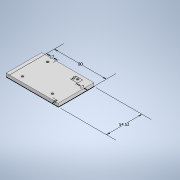
# Autodesk Inventor part: practica 13.2
Saved by Autodesk Inventor 2020.2 (Build 242310000, 310)
## iProperties
Created: 2020-02-28
Part Number: practica 13.2
Material: Genérico
Document SubType Name: Chapa
Designer: Luis Gallardo
Density: 1 g/cm^3
Sheet Metal Rule: Por defecto_mm
Appearance: Valor por defecto
Author: Luis Gallardo
Autodesk Inventor part; units mm, degrees
ref_plane "YZ Plane" through (0, 0, 0) normal (1, 0, 0) x (0, 1, 0)
ref_plane "XZ Plane" through (0, 0, 0) normal (0, 1, 0) x (-1, 0, 0)
ref_plane "XY Plane" through (0, 0, 0) normal (0, 0, 1) x (1, 0, 0)
sketch "Boceto1" plane through (0, 0, 0) normal (0, 1, 0) x (-1, 0, 0)
  line L0 (0, 0) -> (-80, 0)
  line L1 (-80, 0) -> (-80, -54.52)
  line L2 (-80, -54.52) -> (0, -54.52)
  line L3 (0, -54.52) -> (0, 0)
  line L4 (-80, -54.52) -> (-63, -54.52) construction
  line L5 (-63, -54.52) -> (-63, -46.52) construction
  line L6 (-63, 0) -> (-63, -8) construction
  line L7 (0, -54.52) -> (-17, -54.52) construction
  line L8 (-17, -54.52) -> (-17, -46.52) construction
  line L9 (-17, 0) -> (-17, -8) construction
  dimension "d0" = 80
  dimension "d1" = 54.52
  dimension "d2" = 17
  dimension "d3" = 8
  dimension "d6" = 8
  dimension "d7" = 17
  constraints: 20 end point, 6 perpendicular, 4 point on line, 1 horizontal, 1 parallel
  measures "d0" distance of L0.start L0.end
  measures "d1" distance of L0.end L1.end
  measures "d2" distance of L1.end L4.end
  measures "d3" distance of L4.end L5.end
  measures "d6" distance of L6.start L6.end
  measures "d7" distance of L2.end L7.end
extrude "Extrusión1" add sketch "Boceto1" along normal blind 5
hole "Agujero2" at (63, 0, -46.52) direction (0, 1, 0) diameter 3.242 end through all thread size "M4x0.7" class "6H" standard "ANSI Metric M Profile"
hole "Agujero3" at (17, 0, -46.52) at (63, 0, -8) at (17, 0, -8) direction (0, 1, 0) diameter 3.242 end through all thread size "M4x0.7" class "6H" standard "ANSI Metric M Profile"
equation "\"Radio_pliegue\" = Grosor"
equation "\"Anchura_desahogo_plegado\" = Grosor"
equation "\"Profundidad_desahogo_plegado\" = 0.5 * Grosor"
equation "\"Tamaño_destalonado\" = 4 * Grosor"
equation "\"Remanente_mínimo\" = 2 * Grosor"
equation "\"Radiodetransición\" = Radio_pliegue"
equation "\"Tamaño_de_radio_de_Jacobi\" = Radio_pliegue"
equation "\"TamañoSeparación\" = Grosor"
equation "\"Grosor\" = 0.5"
